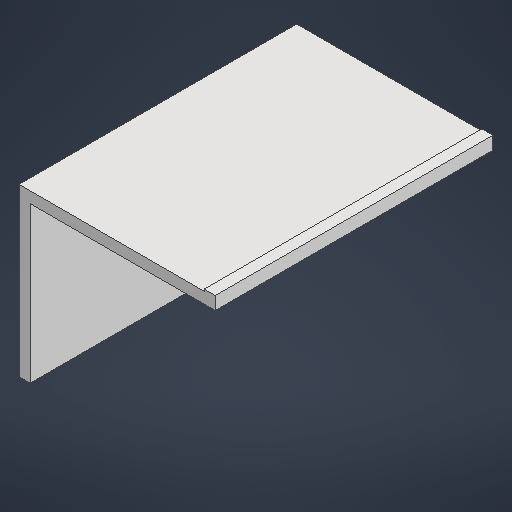
# Autodesk Inventor part: 主体
Saved by Autodesk Inventor 2025 (Build 290162000, 162)
## iProperties
Created: 2025-11-30
Part Number: 主体
Material: 常规
Document SubType Name: Modeling
Designer: XH
Density: 1 g/cm^3
Appearance: 默认
Author: XH
Autodesk Inventor part; units mm, degrees
ref_plane "YZ Plane" through (0, 0, 0) normal (1, 0, 0) x (0, 1, 0)
ref_plane "XZ Plane" through (0, 0, 0) normal (0, 1, 0) x (-1, 0, 0)
ref_plane "XY Plane" through (0, 0, 0) normal (0, 0, 1) x (1, 0, 0)
sketch "草图1" plane through (0, 0, 0) normal (1, 0, 0) x (0, 1, 0)
  line L0 (-22.5, 37.5) -> (22.5, 37.5)
  line L1 (22.5, 37.5) -> (22.5, -37.5)
  line L2 (22.5, -37.5) -> (-22.5, -37.5)
  line L3 (-22.5, -37.5) -> (-22.5, 37.5)
  line L4 (-22.5, 37.5) -> (22.5, -37.5) construction
  line L5 (22.5, 37.5) -> (-22.5, -37.5) construction
  point P0 (0, 0)
  dimension "d2" = 75
  dimension "d3" = 45
  constraints: 12 end point, 2 midpoint, 2 parallel, 1 horizontal, 1 perpendicular
  measures "d2" distance of L2.end L0.start
  measures "d3" distance of L1.end L2.end
extrude "拉伸1" add sketch "草图1" along normal blind 3
sketch "草图2" plane through (3, 0, 0) normal (1, 0, 0) x (0, 0, -1)
  line L0 (37.5, 22.5) -> (-37.5, 22.5) projected
  line L1 (-37.5, 22.5) -> (37.5, 22.5)
  line L2 (37.5, 22.5) -> (37.5, 19.5)
  line L3 (37.5, 19.5) -> (-37.5, 19.5)
  line L4 (-37.5, 19.5) -> (-37.5, 22.5)
  line L5 (37.5, -22.5) -> (37.5, 22.5) projected
  point P0 (0, 0)
  dimension "d4" = 3
  constraints: 8 end point, 2 parallel, 1 collinear, 1 horizontal, 1 perpendicular
  measures "d4" distance between parallel lines of L0 L3
extrude "拉伸2" add sketch "草图2" along normal blind 50
sketch "草图3" plane through (0, 22.5, 37.5) normal (0, 1, 0) x (1, 0, 0)
  line L0 (50, 0) -> (50, 75) projected
  line L1 (0, 75) -> (53, 75) projected
  line L2 (53, 75) -> (50, 75)
  line L3 (50, 75) -> (50, 0)
  line L4 (50, 0) -> (53, 0)
  line L5 (53, 0) -> (53, 75)
  point P0 (0, 37.5)
  constraints: 8 end point, 2 parallel, 1 horizontal, 1 perpendicular
extrude "拉伸3" add sketch "草图3" along normal blind 0.5
